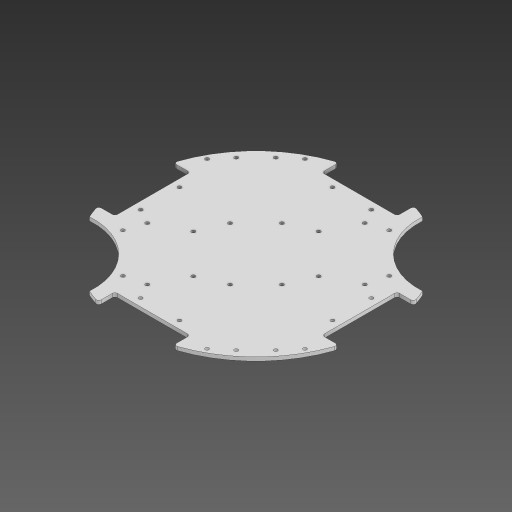
# Autodesk Inventor part: top
Saved by Autodesk Inventor 2023 (Build 270158000, 158)
## iProperties
Created: 2025-06-24
Part Number: top
Material: Типовые
Document SubType Name: Modeling
Designer: daa
Density: 1 g/cm^3
Appearance: По умолчанию
Author: daa
Autodesk Inventor part; units mm, degrees
ref_plane "YZ Plane" through (0, 0, 0) normal (1, 0, 0) x (0, 1, 0)
ref_plane "XZ Plane" through (0, 0, 0) normal (0, 1, 0) x (-1, 0, 0)
ref_plane "XY Plane" through (0, 0, 0) normal (0, 0, 1) x (1, 0, 0)
sketch "Эскиз1" plane through (0, 0, 0) normal (0, 1, 0) x (-1, 0, 0)
  line L0 (-79, -47.2724) -> (-79, 14.7276)
  line L1 (91.5447, -47.2724) -> (91.5447, 14.7276)
  line L2 (-79, -47.2724) -> (-93, -47.2724)
  line L3 (-79, 14.7276) -> (-93, 14.7276)
  line L4 (91.5447, -47.2724) -> (105.5447, -47.2724)
  line L5 (91.5447, 14.7276) -> (105.5447, 14.7276)
  line L6 (-24.7276, -101.5447) -> (37.2724, -101.5447)
  line L7 (-24.7276, 69) -> (37.2724, 69)
  line L8 (-24.7276, 69) -> (-24.7276, 83)
  line L9 (37.2724, 69) -> (37.2724, 83)
  line L10 (37.2724, -101.5447) -> (37.2724, -115.5447)
  line L11 (-24.7276, -101.5447) -> (-24.7276, -115.5447)
  arc A0 (-93, -47.2724) -> (-24.7276, -115.5447) centre (6.2724, -16.2724) ccw
  arc A1 (105.5447, 14.7276) -> (37.2724, 83) centre (6.2724, -16.2724) ccw
  arc A2 (-24.7276, 83) -> (-93, 14.7276) centre (6.2724, -16.2724) ccw
  arc A3 (37.2724, -115.5447) -> (105.5447, -47.2724) centre (6.2724, -16.2724) ccw
  dimension "d29" = 62
  dimension "d31" = 62
  dimension "d33" = 14
  dimension "d34" = 14
  dimension "d35" = 62
  dimension "d36" = 62
  dimension "d39" = 14
  dimension "d40" = 14
  constraints: 24 end point, 8 point on circle, 4 centre point, 4 horizontal, 3 parallel, 3 vertical, 2 point on line, 1 concentric
  measures "d29" distance of L0.start L0.end
  measures "d31" distance of L1.start L1.end
  measures "d33" distance of L0.end L3.end
  measures "d34" distance of L1.end L5.end
  measures "d35" distance of L6.start L6.end
  measures "d36" distance of L7.start L7.end
  measures "d39" distance of L7.start L8.end
  measures "d40" distance of L6.start L11.end
extrude "motor" add sketch "Эскиз1" along normal blind 3
sketch "Эскиз2" plane through (0, 3, 0) normal (0, 1, 0) x (1, 0, 0)
  line L0 (-6.2982, -69) -> (-6.2982, 102)
  line L1 (-88.8109, 16.5) -> (79, 16.5)
  arc A0 (24.7276, -83) -> (93, -14.7276) centre (-6.2724, 16.2724) ccw projected
  line L2 (-6.2982, 16.355) -> (97.7785, 16.355) construction
  line L3 (67.2952, -57.2383) -> (-79.783, 89.8399)
  line L4 (-88.7917, -14.3063) -> (-40.8426, -62.2554)
  line L5 (-101.3809, -25.8032) -> (-48.3479, -78.8362)
  arc A1 (-105.5447, -14.7276) -> (-37.2724, -83) centre (-6.2724, 16.2724) ccw
  arc A2 (-48.3479, -78.8362) -> (-101.3809, -25.8032) centre (-98.035, -75.4903) ccw
  line L6 (24.3631, 98.8485) -> (72.3122, 50.8994)
  line L7 (35.8601, 111.4378) -> (88.8931, 58.4048)
  arc A3 (35.8601, 111.4378) -> (88.8931, 58.4048) centre (85.5471, 108.0918) ccw
  arc A4 (93.0568, 47.3292) -> (24.7845, 115.6015) centre (-6.2155, 16.3292) ccw
  point P0 (0, 0)
  point P1 (-37.2724, -69)
  point P2 (-91.5447, -14.7276)
  point P3 (79.0568, 47.3292)
  point P4 (24.7845, 101.6015)
  dimension "d225" = 75
  dimension "d226" = 17.0315
  constraints: 16 end point, 12 symmetric about line, 9 point on circle, 4 centre point, 2 horizontal, 1 tangent, 1 vertical, 2 other
  measures "d225" distance of L5.start L5.end
  measures "d226" distance between parallel lines of L4 L5
extrude "ball" cut sketch "Эскиз2" against normal blind 3 contours A2 L5 | L5 A1 | A4 L7 | L7 A3
sketch "Эскиз3" plane through (0, 3, 0) normal (0, 1, 0) x (1, 0, 0)
  arc A0 (93, 47.2724) -> (24.7276, 115.5447) centre (-6.2724, 16.2724) ccw projected
  line L0 (-6.2724, 16.2724) -> (97.7276, 16.2724) construction
  line L1 (67.2668, 89.8115) -> (-62.5447, -40)
  circle A1 centre (70.5306, -44.2673) radius 1.5
  circle A2 centre (54.2672, -60.5308) radius 1.5
  circle A3 centre (41.3053, -71.6104) radius 1.5
  circle A4 centre (81.6104, -31.3053) radius 1.5
  arc A5 (24.7276, -83) -> (93, -14.7276) centre (-6.2724, 16.2724) ccw projected
  line L2 (-6.2724, 16.2724) -> (97.7276, 16.2724) construction
  line L3 (-79.8115, 89.8115) -> (67.2668, -57.2668)
  line L4 (-91.5447, 47.2724) -> (-91.5447, -14.7276) projected
  line L5 (-91.5447, 16.2724) -> (79, 16.2724)
  line L6 (24.7276, 101.5447) -> (-37.2724, 101.5447) projected
  line L7 (-6.2724, 101.5447) -> (-6.2724, -69)
  line L8 (-6.2724, 101.5447) -> (-6.2724, -69)
  line L9 (-91.5447, 47.2724) -> (-91.5447, -14.7276) projected
  arc A6 (24.7276, -83) -> (93, -14.7276) centre (-6.2724, 16.2724) ccw projected
  circle A7 centre (-66.812, 93.0753) radius 1.5
  circle A8 centre (-83.0755, 76.8119) radius 1.5
  circle A9 centre (-94.1551, 63.85) radius 1.5
  circle A10 centre (-53.85, 104.1551) radius 1.5
  point P0 (0, 0)
  point P1 (67.2668, -57.2668)
  point P2 (67.2668, -57.2668)
  point P3 (-105.5447, 47.2724)
  point P4 (-79.8115, 89.8115)
  point P5 (-79.8115, 89.8115)
  point P6 (-79.8115, 89.8115)
  dimension "d65" = 3
  dimension "d66" = 3
  dimension "d67" = 3
  dimension "d68" = 3
  dimension "d69" = 23
  dimension "d71" = 57
  dimension "d74" = -12.962
  dimension "d78" = 25.9614
  constraints: 14 end point, 8 centre point, 8 symmetric about line, 4 point on circle, 3 midpoint, 2 horizontal, 2 vertical, 1 point on line, 4 other
  measures "d65" diameter of A1
  measures "d66" diameter of A2
  measures "d67" diameter of A3
  measures "d68" diameter of A4
  measures "d69" distance of A2.centre A1.centre
  measures "d71" distance of A3.centre A4.centre
  measures "d74" vertical distance of A1.centre A4.centre
  measures "d78" vertical distance of A4.centre point (67.267, -57.267)
extrude "hand_mount" cut sketch "Эскиз3" against normal blind 10
sketch "Эскиз5" plane through (0, 3, 0) normal (0, 1, 0) x (1, 0, 0)
  circle A0 centre (-6.2982, 16.355) radius 104
  arc A1 (-105.5447, -14.7276) -> (-99.04, -30.7083) centre (-6.2982, 16.355) ccw projected
  line L0 (-6.2982, 16.355) -> (97.7018, 16.355) construction
  line L1 (66.7419, 90.3898) -> (-80.333, -56.685)
  circle A2 centre (-45.4039, -54.2829) radius 1.5
  arc A3 (-53.253, -76.4953) -> (-99.04, -30.7083) centre (-88.8109, -66.2662) ccw projected
  line L2 (-63.2054, -39.5574) -> (-61.6674, -38.0194)
  line L3 (-61.6674, -38.0194) -> (-45.3883, -38.0194) construction
  line L4 (-61.6674, -38.0194) -> (-45.4039, -54.2829)
  circle A4 centre (-77.9308, -21.756) radius 1.5
  arc A5 (24.7276, -83) -> (93, -14.7276) centre (-6.2724, 16.2724) ccw projected
  line L5 (-6.2982, 16.355) -> (97.7785, 16.355) construction
  line L6 (67.2952, -57.2383) -> (-79.783, 89.8399)
  arc A6 (-37.2724, 115.5447) -> (-105.5447, 47.2724) centre (-6.2724, 16.2724) ccw projected
  circle A7 centre (64.3397, 55.4608) radius 1.5
  circle A8 centre (31.8128, 87.9877) radius 1.5
  point P0 (0, 0)
  point P1 (-99.6577, -29.5007)
  point P2 (-54.9732, -51.2992)
  point P3 (-73.8439, -32.4285)
  dimension "d119" = 208
  dimension "d126" = 3
  dimension "d130" = 2.175
  dimension "d133" = 23
  constraints: 14 end point, 4 centre point, 4 point on circle, 3 horizontal, 3 symmetric about line, 2 point on line, 1 coincident, 7 other
  measures "d126" diameter of A2
  measures "d130" distance of L2.start L2.end
  measures "d133" distance of L2.end L4.end
extrude "Выдавливание5" cut sketch "Эскиз5" against normal blind 10 contours A2 | A4 | A7 | A8
sketch "Эскиз6" plane through (0, 3, 0) normal (0, 1, 0) x (1, 0, 0)
  circle A0 centre (-22.2724, 95.2947) radius 1.5
  circle A1 centre (9.7276, 95.2947) radius 1.5
  line L0 (24.7276, 115.5447) -> (24.7276, 101.5447) projected
  line L1 (24.7276, 101.5447) -> (-37.2724, 101.5447) projected
  circle A2 centre (-22.2724, -62.75) radius 1.5
  circle A3 centre (9.7276, -62.75) radius 1.5
  circle A4 centre (-85.2947, 32.2724) radius 1.5
  circle A5 centre (-85.2947, 0.2724) radius 1.5
  circle A6 centre (72.75, 32.2724) radius 1.5
  circle A7 centre (72.75, 0.2724) radius 1.5
  point P0 (0, 0)
  point P1 (24.7276, -69)
  point P2 (-37.2724, -69)
  point P3 (-91.5447, -14.7276)
  point P4 (-91.5447, 47.2724)
  point P5 (79, 47.2724)
  point P6 (79, -14.7276)
  dimension "d135" = 3
  dimension "d136" = 3
  dimension "d137" = 32
  dimension "d138" = 15
  dimension "d139" = 6.25
  dimension "d140" = 3
  dimension "d141" = 3
  dimension "d142" = 6.25
  dimension "d143" = 32
  dimension "d144" = 15
  dimension "d145" = 6.25
  dimension "d146" = 6.25
  dimension "d147" = 3
  dimension "d148" = 3
  dimension "d149" = 32
  dimension "d150" = 15
  dimension "d151" = 6.25
  dimension "d152" = 6.25
  dimension "d153" = 3
  dimension "d154" = 3
  dimension "d155" = 32
  dimension "d156" = 15
  dimension "d157" = 6.25
  dimension "d158" = 6.25
  constraints: 8 centre point
  measures "d135" diameter of A0
  measures "d136" diameter of A1
  measures "d137" distance of A1.centre A0.centre
  measures "d138" distance from line of L0 A1.centre
  measures "d139" distance from line of L1 A1.centre
  measures "d140" diameter of A2
  measures "d141" diameter of A3
  measures "d142" distance from line of L1 A0.centre
  measures "d143" distance of A2.centre A3.centre
  measures "d144" horizontal distance of point (24.728, -69) A3.centre
  measures "d145" vertical distance of point (24.728, -69) A3.centre
  measures "d146" vertical distance of point (-37.272, -69) A2.centre
  measures "d147" diameter of A4
  measures "d148" diameter of A5
  measures "d149" distance of A5.centre A4.centre
  measures "d150" vertical distance of A5.centre point (-91.545, -14.728)
  measures "d151" horizontal distance of A5.centre point (-91.545, -14.728)
  measures "d152" horizontal distance of A4.centre point (-91.545, 47.272)
  measures "d153" diameter of A6
  measures "d154" diameter of A7
  measures "d155" distance of A7.centre A6.centre
  measures "d156" vertical distance of point (79, 47.272) A6.centre
  measures "d157" horizontal distance of point (79, -14.728) A7.centre
  measures "d158" horizontal distance of point (79, 47.272) A6.centre
extrude "Выдавливание6" cut sketch "Эскиз6" against normal blind 10
fillet "Сопряжение1" radius 2 16 edges at (93, 1.5, -47.2724) (24.7276, 1.5, -115.5447) (24.7276, 1.5, -101.5447) (-37.2724, 1.5, -101.5447) (-37.2724, 1.5, -115.5447) (-105.5447, 1.5, -47.2724) (-91.5447, 1.5, -47.2724) (-91.5447, 1.5, 14.7276) (-105.5447, 1.5, 14.7276) (-37.2724, 1.5, 83) (-37.2724, 1.5, 69) (24.7276, 1.5, 69) (24.7276, 1.5, 83) (93, 1.5, 14.7276) (79, 1.5, 14.7276) (79, 1.5, -47.2724)
sketch "Эскиз7" plane through (0, 3, 0) normal (0, 1, 0) x (1, 0, 0)
  line L0 (-17.5157, 48.87) -> (26.3249, 5.0294)
  line L1 (26.3249, 5.0294) -> (4.9703, -16.3253)
  line L2 (4.9703, -16.3253) -> (-38.8704, 27.5154)
  line L3 (-38.8704, 27.5154) -> (-17.5157, 48.87)
  circle A0 centre (-6.2724, 16.2724) radius 104
  arc A1 (-39.9194, 114.679) -> (-104.679, 49.9194) centre (-6.2724, 16.2724) ccw projected
  circle A2 centre (-17.5157, 48.87) radius 1.5
  circle A3 centre (-38.8704, 27.5154) radius 1.5
  circle A4 centre (4.9703, -16.3253) radius 1.5
  circle A5 centre (26.3249, 5.0294) radius 1.5
  line L4 (11.3776, -15.2276) -> (11.3776, -22.2276)
  dimension "d165" = 62
  dimension "d166" = 30.2
  dimension "d167" = 208
  dimension "d168" = 32.598
  dimension "d170" = -11.243
  dimension "d171" = 3
  dimension "d172" = 3
  dimension "d173" = 3
  dimension "d174" = 3
  constraints: 10 end point, 5 centre point, 3 coincident, 2 parallel, 1 concentric, 1 perpendicular, 1 point on line
  measures "d165" distance of L1.end L2.end
  measures "d166" distance of L0.end L1.end
  measures "d167" diameter of A0
  measures "d168" horizontal distance of A1.centre L2.end
  measures "d170" vertical distance of L0.end A1.centre
  measures "d171" diameter of A2
  measures "d172" diameter of A3
  measures "d173" diameter of A4
  measures "d174" diameter of A5
extrude "Выдавливание7" cut sketch "Эскиз7" against normal through all contours L3 A2 L0 | L0 A2 L3 | A5 L1 L0 | L0 L1 A5 | A3 L2 L3 | L3 L2 A3 | A4 L2 L1 | L1 L2 A4
sketch "Эскиз8" plane through (0, 3, 0) normal (0, 1, 0) x (1, 0, 0)
  line L0 (-16.0658, -25.5526) -> (-48.0977, 6.4794)
  line L1 (-48.0977, 6.4794) -> (3.5211, 58.0981)
  line L2 (3.5211, 58.0981) -> (35.553, 26.0662)
  line L3 (35.553, 26.0662) -> (-16.0658, -25.5526)
  circle A0 centre (-6.2724, 16.2724) radius 104
  arc A1 (-39.9194, 114.679) -> (-104.679, 49.9194) centre (-6.2724, 16.2724) ccw projected
  circle A2 centre (-16.0658, -25.5526) radius 1.5
  circle A3 centre (-48.0977, 6.4794) radius 1.5
  circle A4 centre (35.553, 26.0662) radius 1.5
  circle A5 centre (3.5211, 58.0981) radius 1.5
  point P0 (0, 0)
  dimension "d198" = 73
  dimension "d199" = 45.3
  dimension "d200" = 208
  dimension "d201" = -9.793
  dimension "d202" = 9.7934
  dimension "d203" = 3
  dimension "d204" = 3
  dimension "d205" = 3
  dimension "d206" = 3
  constraints: 8 end point, 5 centre point, 4 coincident, 2 parallel, 1 concentric, 1 perpendicular
  measures "d198" distance of L0.end L1.end
  measures "d199" distance of L1.end L2.end
  measures "d200" diameter of A0
  measures "d201" vertical distance of A0.centre L0.end
  measures "d202" horizontal distance of L0.start A1.centre
  measures "d203" diameter of A2
  measures "d204" diameter of A3
  measures "d205" diameter of A4
  measures "d206" diameter of A5
extrude "Выдавливание8" cut sketch "Эскиз8" against normal through all contours L3 A2 L0 | L0 A2 L3 | A3 L1 L0 | L0 L1 A3 | A4 L2 L3 | L3 L2 A4 | A5 L2 L1 | L1 L2 A5
sketch "Эскиз9" plane through (0, 3, 0) normal (0, 1, 0) x (1, 0, 0)
  circle A0 centre (-6.2724, 16.2724) radius 104
  arc A1 (-39.9194, 114.679) -> (-104.679, 49.9194) centre (-6.2724, 16.2724) ccw projected
  arc A2 (-102.7866, -14.7276) -> (-104.679, -17.3747) centre (-102.7866, -16.7276) ccw projected
  line L0 (-104.676, -17.3763) -> (-104.676, 49.9282)
  arc A3 (-104.676, -17.3763) -> (-99.7731, -29.235) centre (-6.2982, 16.355) ccw projected
  line L1 (-51.7797, -77.2284) -> (-99.7731, -29.235)
  circle A4 centre (-29.1928, -50.38) radius 1.5
  circle A5 centre (-73.0334, -6.5394) radius 1.5
  arc A6 (27.3747, -82.1343) -> (92.1343, -17.3747) centre (-6.2724, 16.2724) ccw projected
  line L2 (-6.2982, 16.355) -> (97.7785, 16.355) construction
  line L3 (67.2952, -57.2383) -> (-79.8115, 89.8115)
  circle A7 centre (60.3995, 39.2469) radius 1.5
  circle A8 centre (16.542, 83.0706) radius 1.5
  point P0 (72.4394, -51.7016)
  dimension "d209" = 208
  dimension "d216" = 3
  dimension "d217" = 3
  dimension "d218" = 62
  dimension "d219" = 66.735
  dimension "d220" = 31.6426
  dimension "d221" = 75.4832
  constraints: 8 end point, 5 centre point, 3 point on circle, 2 symmetric about line, 1 concentric, 1 horizontal, 1 vertical, 2 other
  measures "d209" diameter of A0
  measures "d216" diameter of A4
  measures "d217" diameter of A5
  measures "d218" distance of A5.centre A4.centre
  measures "d219" vertical distance of L2.start A4.centre
  measures "d220" distance from line of L0 A5.centre
  measures "d221" distance from line of L0 A4.centre
extrude "Выдавливание9" cut sketch "Эскиз9" against normal blind 10 contours A4 | A5 | A7 | A8
